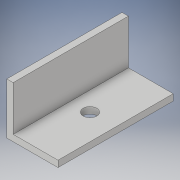
# Autodesk Inventor part: uchannel
Saved by Autodesk Inventor 2017 (Build 210142000, 142)
## iProperties
Created: 2018-10-17
Part Number: uchannel
Material: Generic
Document SubType Name: Modeling
Designer: ddeboer
Density: 1 g/cm^3
Appearance: Default
Author: ddeboer
Autodesk Inventor part; units mm, degrees
ref_plane "YZ Plane" through (0, 0, 0) normal (1, 0, 0) x (0, 1, 0)
ref_plane "XZ Plane" through (0, 0, 0) normal (0, 1, 0) x (-1, 0, 0)
ref_plane "XY Plane" through (0, 0, 0) normal (0, 0, 1) x (1, 0, 0)
sketch "Sketch1" plane through (0, 0, 0) normal (0, 0, 1) x (1, 0, 0)
  line L0 (0, 0) -> (25.4, 0)
  line L1 (0, 0) -> (0, 25.4)
  line L2 (3.175, 4.953) -> (3.175, 25.4)
  line L3 (3.175, 25.4) -> (0, 25.4)
  line L4 (4.953, 3.175) -> (25.4, 3.175)
  line L5 (25.4, 3.175) -> (25.4, 0)
  line L6 (3.175, 4.953) -> (3.175, 3.175)
  line L7 (3.175, 3.175) -> (4.953, 3.175)
  dimension "d6" = 25.4
  dimension "d7" = 25.4
  constraints: 16 end point, 3 perpendicular, 3 vertical, 2 horizontal
  measures "d6" distance of L0.start L0.end
  measures "d7" distance of L0.start L1.end
extrude "Extrusion1" add sketch "Sketch1" along normal blind 57.15
sketch "Sketch2" plane through (3.175, 3.175, 0) normal (0, 1, 0) x (1, 0, 0)
  circle A0 centre (9.525, -28.575) radius 3.076
  line L0 (22.225, 0) -> (22.225, -57.15) projected
  line L1 (22.225, 0) -> (0, 0) projected
  line L2 (22.225, -57.15) -> (0, -57.15) projected
  point P0 (-3.175, 0)
  dimension "d8" = 12.7
  dimension "d9" = 28.575
  dimension "d10" = 28.575
  constraints: 1 centre point
  measures "d8" distance from line of A0.centre L0
  measures "d9" distance from line of A0.centre L1
  measures "d10" distance from line of A0.centre L2
hole "Hole1" at (12.7, 3.175, 28.575) direction (0, -1, 0) diameter 6.7564 depth 25.4 tip angle 118 clearance for "Flat Head Machine Screw (82)" size "1/4" standard "Ansi Unified Screw Threads"
body "Solid1"
